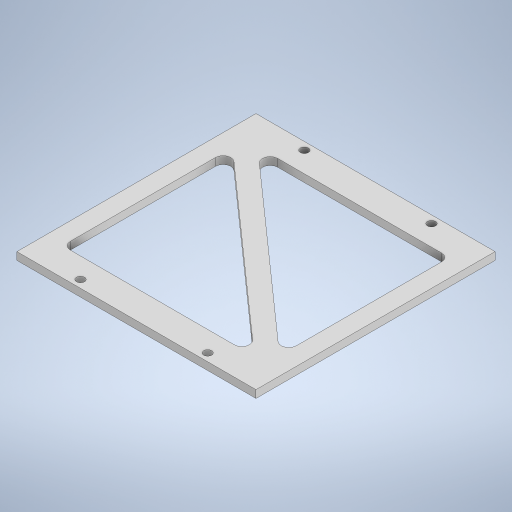
# Autodesk Inventor part: FrontPanel
Saved by Autodesk Inventor 2023 (Build 270158000, 158)
## iProperties
Created: 2022-07-23
Part Number: FrontPanel
Material: Generic
Document SubType Name: Modeling
Designer: Aditya Bansal
Density: 1 g/cm^3
Appearance: Default
Author: Aditya Bansal
Autodesk Inventor part; units mm, degrees
ref_plane "YZ Plane" through (0, 0, 0) normal (1, 0, 0) x (0, 1, 0)
ref_plane "XZ Plane" through (0, 0, 0) normal (0, 1, 0) x (-1, 0, 0)
ref_plane "XY Plane" through (0, 0, 0) normal (0, 0, 1) x (1, 0, 0)
sketch "Sketch1" plane through (0, 0, 0) normal (0, 1, 0) x (-1, 0, 0)
  line L0 (0, 0) -> (94, 0)
  line L1 (94, -94) -> (0, -94)
  line L2 (0, -94) -> (0, 0)
  line L3 (94, 0) -> (0, 0) construction
  line L4 (0, 0) -> (0, -6) construction
  line L5 (0, -6) -> (94, -6) construction
  line L6 (94, -6) -> (94, 0) construction
  line L7 (0, -94) -> (94, -94) construction
  line L8 (94, -94) -> (94, -88) construction
  line L9 (94, -88) -> (0, -88) construction
  line L10 (0, -88) -> (0, -94) construction
  line L11 (94, 0) -> (94, -94)
  circle A0 centre (72, -3) radius 1.6
  circle A1 centre (22, -3) radius 1.6
  circle A2 centre (72, -91) radius 1.6
  circle A3 centre (22, -91) radius 1.6
  line L12 (87, -11) -> (87, -77.7604)
  line L13 (87, -77.7604) -> (11.6418, -11)
  line L14 (11.6418, -11) -> (87, -11)
  line L15 (7, -16.2396) -> (82.3582, -83)
  line L16 (82.3582, -83) -> (7, -83)
  line L17 (7, -83) -> (7, -16.2396)
  line L18 (82.3582, -83) -> (87, -77.7604) construction
  line L19 (11.6418, -11) -> (7, -16.2396) construction
  point P0 (47, -6)
  dimension "d0" = 94
  dimension "d1" = 6
  dimension "d2" = 3
  dimension "d3" = 3.2
  dimension "d6" = 94
  dimension "d7" = 3
  dimension "d10" = 25
  dimension "d11" = 50
  dimension "d12" = 7
  dimension "d13" = 5
  dimension "d14" = 7
  dimension "d15" = 5
  dimension "d16" = 7
  constraints: 41 end point, 8 parallel, 6 perpendicular, 4 centre point, 3 equal radius, 3 horizontal, 2 collinear, 2 horizontal alignment, 2 vertical alignment, 1 midpoint, 1 point on line, 1 vertical
  measures "d0" distance of L0.end L1.start
  measures "d1" distance between parallel lines of L1 L9
  measures "d2" distance from line of L5 A0.centre
  measures "d3" diameter of A0
  measures "d6" distance of L1.start L1.end
  measures "d7" distance from line of L9 A2.centre
  measures "d10" horizontal distance of point (47, -6) A0.centre
  measures "d11" distance of A1.centre A0.centre
  measures "d12" distance between parallel lines of L2 L17
  measures "d13" distance between parallel lines of L5 L14
  measures "d14" distance between parallel lines of L11 L12
  measures "d15" distance between parallel lines of L9 L16
  measures "d16" distance between parallel lines of L13 L15
extrude "Extrusion1" add sketch "Sketch1" along normal blind 3
fillet "Fillet1" radius 3 6 edges at (-87, 1.5, -77.7604) (-82.3582, 1.5, -83) (-7, 1.5, -16.2396) (-11.6418, 1.5, -11) (-87, 1.5, -11) (-7, 1.5, -83)
equation "\"d11\" = 2 * d10"
equation "\"d13\" = d15"
equation "\"d14\" = d12"
body "Solid1"
